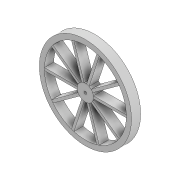
# Autodesk Inventor part: PoleaX
Saved by Autodesk Inventor 2021 (Build 250183000, 183)
## iProperties
Created: 2022-02-09
Part Number: PoleaX
Material: Generic
Document SubType Name: Modeling
Designer: Santiago
Density: 1 g/cm^3
Appearance: Default
Author: Santiago
Autodesk Inventor part; units mm, degrees
ref_plane "YZ Plane" through (0, 0, 0) normal (1, 0, 0) x (0, 1, 0)
ref_plane "XZ Plane" through (0, 0, 0) normal (0, 1, 0) x (-1, 0, 0)
ref_plane "XY Plane" through (0, 0, 0) normal (0, 0, 1) x (1, 0, 0)
sketch "Sketch1" plane through (0, 0, 0) normal (0, 0, 1) x (1, 0, 0)
  circle A0 centre (0, 0) radius 225
  circle A1 centre (0, 0) radius 6.35
  circle A2 centre (0, 0) radius 40
  circle A3 centre (0, 0) radius 200
  line L0 (-40, 0) -> (-200, 0)
  line L1 (-200, 0) -> (-39.4928, 0)
  line L2 (-39.4928, 0) -> (-39.4928, 6.35)
  line L3 (-39.4928, 6.35) -> (-200, 6.35)
  line L4 (-200, 6.35) -> (-200, 0)
  line L5 (-39.4928, 0) -> (-39.4928, -6.35)
  line L6 (-39.4928, -6.35) -> (-200, -6.35)
  line L7 (-200, -6.35) -> (-200, 0)
  line L8 (-32.3607, -23.5114) -> (-161.8034, -117.5571)
  line L9 (-161.8034, -117.5571) -> (-31.9503, -23.2133)
  line L10 (-31.9503, -23.2133) -> (-35.6827, -18.076)
  line L11 (-35.6827, -18.076) -> (-165.5358, -112.4198)
  line L12 (-165.5358, -112.4198) -> (-161.8034, -117.5571)
  line L13 (-28.2179, -28.3505) -> (-158.071, -122.6943)
  line L14 (-31.9503, -23.2133) -> (-28.2179, -28.3505)
  line L15 (-158.071, -122.6943) -> (-161.8034, -117.5571)
  line L16 (-12.3607, -38.0423) -> (-61.8034, -190.2113)
  line L17 (-61.8034, -190.2113) -> (-12.2039, -37.5598)
  line L18 (-12.2039, -37.5598) -> (-18.2431, -35.5976)
  line L19 (-18.2431, -35.5976) -> (-67.8426, -188.249)
  line L20 (-67.8426, -188.249) -> (-61.8034, -190.2113)
  line L21 (-6.1647, -39.5221) -> (-55.7642, -192.1736)
  line L22 (-12.2039, -37.5598) -> (-6.1647, -39.5221)
  line L23 (-55.7642, -192.1736) -> (-61.8034, -190.2113)
  line L24 (12.3607, -38.0423) -> (61.8034, -190.2113)
  line L25 (61.8034, -190.2113) -> (12.2039, -37.5598)
  line L26 (12.2039, -37.5598) -> (6.1647, -39.5221)
  line L27 (6.1647, -39.5221) -> (55.7642, -192.1736)
  line L28 (55.7642, -192.1736) -> (61.8034, -190.2113)
  line L29 (18.2431, -35.5976) -> (67.8426, -188.249)
  line L30 (12.2039, -37.5598) -> (18.2431, -35.5976)
  line L31 (67.8426, -188.249) -> (61.8034, -190.2113)
  line L32 (32.3607, -23.5114) -> (161.8034, -117.5571)
  line L33 (161.8034, -117.5571) -> (31.9503, -23.2133)
  line L34 (31.9503, -23.2133) -> (28.2179, -28.3505)
  line L35 (28.2179, -28.3505) -> (158.071, -122.6943)
  line L36 (158.071, -122.6943) -> (161.8034, -117.5571)
  line L37 (35.6827, -18.076) -> (165.5358, -112.4198)
  line L38 (31.9503, -23.2133) -> (35.6827, -18.076)
  line L39 (165.5358, -112.4198) -> (161.8034, -117.5571)
  line L40 (40, 0) -> (200, 0)
  line L41 (200, 0) -> (39.4928, 0)
  line L42 (39.4928, 0) -> (39.4928, -6.35)
  line L43 (39.4928, -6.35) -> (200, -6.35)
  line L44 (200, -6.35) -> (200, 0)
  line L45 (39.4928, 6.35) -> (200, 6.35)
  line L46 (39.4928, 0) -> (39.4928, 6.35)
  line L47 (200, 6.35) -> (200, 0)
  line L48 (32.3607, 23.5114) -> (161.8034, 117.5571)
  line L49 (161.8034, 117.5571) -> (31.9503, 23.2133)
  line L50 (31.9503, 23.2133) -> (35.6827, 18.076)
  line L51 (35.6827, 18.076) -> (165.5358, 112.4198)
  line L52 (165.5358, 112.4198) -> (161.8034, 117.5571)
  line L53 (28.2179, 28.3505) -> (158.071, 122.6943)
  line L54 (31.9503, 23.2133) -> (28.2179, 28.3505)
  line L55 (158.071, 122.6943) -> (161.8034, 117.5571)
  line L56 (12.3607, 38.0423) -> (61.8034, 190.2113)
  line L57 (61.8034, 190.2113) -> (12.2039, 37.5598)
  line L58 (12.2039, 37.5598) -> (18.2431, 35.5976)
  line L59 (18.2431, 35.5976) -> (67.8426, 188.249)
  line L60 (67.8426, 188.249) -> (61.8034, 190.2113)
  line L61 (6.1647, 39.5221) -> (55.7642, 192.1736)
  line L62 (12.2039, 37.5598) -> (6.1647, 39.5221)
  line L63 (55.7642, 192.1736) -> (61.8034, 190.2113)
  line L64 (-12.3607, 38.0423) -> (-61.8034, 190.2113)
  line L65 (-61.8034, 190.2113) -> (-12.2039, 37.5598)
  line L66 (-12.2039, 37.5598) -> (-6.1647, 39.5221)
  line L67 (-6.1647, 39.5221) -> (-55.7642, 192.1736)
  line L68 (-55.7642, 192.1736) -> (-61.8034, 190.2113)
  line L69 (-18.2431, 35.5976) -> (-67.8426, 188.249)
  line L70 (-12.2039, 37.5598) -> (-18.2431, 35.5976)
  line L71 (-67.8426, 188.249) -> (-61.8034, 190.2113)
  line L72 (-32.3607, 23.5114) -> (-161.8034, 117.5571)
  line L73 (-161.8034, 117.5571) -> (-31.9503, 23.2133)
  line L74 (-31.9503, 23.2133) -> (-28.2179, 28.3505)
  line L75 (-28.2179, 28.3505) -> (-158.071, 122.6943)
  line L76 (-158.071, 122.6943) -> (-161.8034, 117.5571)
  line L77 (-35.6827, 18.076) -> (-165.5358, 112.4198)
  line L78 (-31.9503, 23.2133) -> (-35.6827, 18.076)
  line L79 (-165.5358, 112.4198) -> (-161.8034, 117.5571)
  point P0 (200, 0)
  point P1 (200, 0)
  point P2 (199.8992, -6.35)
  point P3 (165.4543, -112.3605)
  point P4 (157.9894, -122.635)
  point P5 (67.8114, -188.1531)
  point P6 (55.733, -192.0777)
  point P7 (-55.733, -192.0777)
  point P8 (-67.8114, -188.1531)
  point P9 (-157.9894, -122.635)
  point P10 (-165.4543, -112.3605)
  point P11 (-199.8992, -6.35)
  point P12 (-199.8992, 6.35)
  point P13 (-165.4543, 112.3605)
  point P14 (-157.9894, 122.635)
  point P15 (-67.8114, 188.1531)
  point P16 (-55.733, 192.0777)
  point P17 (55.733, 192.0777)
  point P18 (67.8114, 188.1531)
  point P19 (157.9894, 122.635)
  point P20 (165.4543, 112.3605)
  point P21 (199.8992, 6.35)
  dimension "d4" = 80
  dimension "d5" = 400
  dimension "d0" = 450
  dimension "d1" = 12.7
  dimension "d8" = 360
  constraints: 160 end point, 4 coincident, 2 centre point, 2 horizontal, 2 parallel, 2 symmetric about line, 1 perpendicular, 158 other
  measures "d0" diameter of A0
  measures "d1" diameter of A1
extrude "Extrusion2" add sketch "Sketch1" along normal blind 45 contours A0 | L40 A3 L43 A2 | A2 L45 A3 L40 | L46 L42 A2 L38 L34 L30 L26 L22 L18 L14 L10 L5 L2 L78 L74 L70 L66 L62 L58 L54 L50 | A2 L48 A3 L51 | L37 A3 L32 A2 | A2 L53 A3 L48 | L32 A3 L35 A2 | A2 L56 A3 L59 | L29 A3 L24 A2 | A2 L61 A3 L56 | L24 A3 L27 A2 | A2 L64 A3 L67 | L21 A3 L16 A2 | A2 L69 A3 L64 | L16 A3 L19 A2 | A2 L72 A3 L75 | L13 A3 L8 A2 | A2 L77 A3 L72 | L8 A3 L11 A2 | A2 L0 A3 L3 | L6 A3 L0 A2
body "Solid2"
